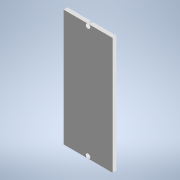
# Autodesk Inventor part: battery_case_top
Saved by Autodesk Inventor 2022 (Build 260153000, 153)
## iProperties
Created: 2022-10-11
Part Number: battery_case_top
Material: Типовые
Document SubType Name: Modeling
Designer: korsh624
Density: 1 g/cm^3
Appearance: По умолчанию
Author: korsh624
Autodesk Inventor part; units mm, degrees
ref_plane "YZ Plane" through (0, 0, 0) normal (1, 0, 0) x (0, 1, 0)
ref_plane "XZ Plane" through (0, 0, 0) normal (0, 1, 0) x (-1, 0, 0)
ref_plane "XY Plane" through (0, 0, 0) normal (0, 0, 1) x (1, 0, 0)
sketch "Эскиз1" plane through (0, 0, 0) normal (0, 0, 1) x (1, 0, 0)
  circle A0 centre (0, 98.9661) radius 2 projected
  circle A1 centre (0, -0.7112) radius 2 projected
  line L0 (-22, 101.1274) -> (22, 101.1274) projected
  line L1 (22, 101.1274) -> (22, -2.8726) projected
  line L2 (22, -2.8726) -> (-22, -2.8726) projected
  line L3 (-22, -2.8726) -> (-22, 101.1274) projected
  line L4 (21.7, 100.8274) -> (-21.7, 100.8274)
  line L5 (-21.7, 100.8274) -> (-21.7, -2.5726)
  line L6 (-21.7, -2.5726) -> (21.7, -2.5726)
  line L7 (21.7, -2.5726) -> (21.7, 100.8274)
  point P0 (0, 0)
  point P1 (-0.7318, -2.5726)
  point P2 (0.7318, -2.5726)
  point P3 (0.7318, 100.8274)
  point P4 (-0.7318, 100.8274)
  dimension "d0" = 0.3
  dimension "d1" = 0.3
  dimension "d2" = 0.3
  dimension "d3" = 0.3
  constraints: 8 end point, 2 parallel, 1 horizontal, 1 perpendicular
  measures "d0" distance between parallel lines of L4 L0
  measures "d1" distance between parallel lines of L7 L1
  measures "d2" distance between parallel lines of L6 L2
  measures "d3" distance between parallel lines of L5 L3
extrude "Выдавливание1" add sketch "Эскиз1" along normal blind 3.5 contours A0 L4 L7 L6 A1 L5
equation "\"d0\" = d1"
equation "\"d2\" = d0"
equation "\"d3\" = d0"
